microwave foot_v1 (Autodesk Fusion 360 design; units mm, degrees)
Autodesk Fusion 360 part; units mm, degrees
sketch "Sketch1" plane through (0, 0, 0) normal (0, 1, 0) x (1, 0, 0)
  line L0 (0, 0) -> (7.5, 0)
  line L1 (7.5, 0) -> (9, -8)
  line L2 (9, -8) -> (4.35, -8)
  line L3 (3.85, -8.5) -> (3.85, -16)
  line L4 (3.85, -16) -> (0, -16)
  line L5 (0, -16) -> (0, 0)
  arc A0 (4.35, -8) -> (3.85, -8.5) centre (4.35, -8.5) ccw
  point P0 (3.85, -8)
  dimension "d1" = 7.5
  dimension "d2" = 8
  dimension "d3" = 3.85
  dimension "d4" = 8
  dimension "d5" = 0.5
  constraint coincident L0.start L5.end
  constraint horizontal L0
  constraint horizontal L2
  constraint perpendicular L2 L3
  constraint perpendicular L3 L4
  constraint perpendicular L0 L5
  constraint coincident P0 L2
  constraint coincident P0 L3
  constraint tangent L2 A0
  constraint tangent L3 A0
  measures "d1" distance of L0.start L0.end
  measures "d2" vertical distance of L0.end L1.end
  measures "d3" distance of L3 L5
  measures "d4" distance of P0 L3.end
  measures "d5" radius of A0
revolve "Revolve1" add sketch "Sketch1" angle 360 about axis through (0, 0, 16) along (0, 0, -1)
chamfer "Chamfer1" distance 1 angle 45 1 edges at (-3.5895, -1.3922, 16)
